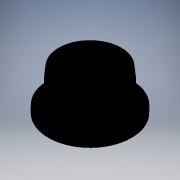
# Autodesk Inventor part: 706368 GPN
Saved by Autodesk Inventor 2017.3 (Build 213256000, 256)
## iProperties
Part Number: 706368 GPN
Material: Generic
Catalog Web Link: www.cadenas.de
Description: GPN-Plug
Vendor: FESTO
Document SubType Name: Modeling
Designer: partserver
Manufacturer: FESTO
Mass: 1.16952 g
Surface Area: 14.5149 cm^2
Volume: 1.16952 cm^3
Density: 1 g/cm^3
Appearance: PSOLRGB-0-0-0
Category: PARTsolutions
Company: FESTO
Title: 706368 GPN
Author: Cadenas PARTsolutions
Comments: Plug
PSOL_IDENT_0: {$CADENAS_DATA\23d-libs\festo\parts\e\eamm\parts\eamm_u_gpn.prj},157 {VTYP=3D},{NB=706368 GPN},{LINA=
PSOL_IDENT_1: 706368 GPN},{NN=GPN},{DATE=27.10.2020 09:44:40},{GEOMDATE=08.01.2020 14:15:00},{VERSION=},{LINEID=10
PSOL_IDENT_2: },{WBVAR=},{WBNUMERIC=}  {NB=706368 GPN},{LINA=706368 GPN},{KT=DUMMY},{TNR=706368},{TYP=GPN}
NB: 706368 GPN
NN: GPN
NT: Plug
NBSYN: $TNR. $TYP.
LINA: 706368 GPN
CATALOG: Festo
TNR: 706368
TYP: GPN
SUPPLIER: FESTO
ARTICLENO: 706368 GPN
BOMINFO: 706368 GPN
CREATOR: CADENAS GmbH
Autodesk Inventor part; units mm, degrees
sketch "Sketch_1" plane through (0, 0, 0) normal (1, 0, 0) x (0, 1, 0)
  line L0 (0, -8) -> (0, 2)
  line L1 (0, 2) -> (9.8, 2)
  arc A0 (10, 1.8) -> (9.8, 2) centre (9.8, 1.8) ccw
  line L2 (10, 1.8) -> (10, 0)
  line L3 (10, 0) -> (7.7314, 0)
  arc A1 (7.7314, 0) -> (7.5334, -0.2281) centre (7.7314, -0.2) ccw
  arc A2 (7.5, -8) -> (7.5334, -0.2281) centre (-19.0167, -4) ccw
  line L4 (7.5, -8) -> (5.8, -8)
  line L5 (5.8, -8) -> (5.8, 0.5)
  arc A3 (5.8, 0.5) -> (5.3, 1) centre (5.3, 0.5) ccw
  line L6 (5.3, 1) -> (0, 1)
  line L7 (0, 1) -> (0, 2)
  constraints: 16 end point, 8 point on circle, 4 centre point
revolve "Revolution1" add sketch "Sketch_1" angle 360 about axis through (0, 0, -8) along (0, 0, -1)
ref_plane "ANBAU_XY" through (0, 0, 0) normal (0, 0, 1) x (1, 0, 0)
ref_plane "ANBAU_YZ" through (0, 0, 0) normal (1, 0, 0) x (0, 1, 0)
ref_plane "ANBAU_ZX" through (0, 0, 0) normal (0, 1, 0) x (0, 0, 1)
body "Solid1"
